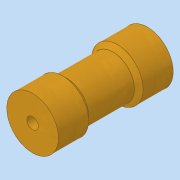
# Autodesk Inventor part: ShaftCoupler
Saved by Autodesk Inventor 2017 (Build 210142000, 142)
## iProperties
Created: 2017-03-06
Part Number: ShaftCoupler
Material: Brass, Soft Yellow, Welded
Document SubType Name: Modeling
Designer: techn
Density: 8.5 g/cm^3
Appearance: Weld - Brass
Author: techn
Autodesk Inventor part; units mm, degrees
ref_plane "YZ Plane" through (0, 0, 0) normal (1, 0, 0) x (0, 1, 0)
ref_plane "XZ Plane" through (0, 0, 0) normal (0, 1, 0) x (-1, 0, 0)
ref_plane "XY Plane" through (0, 0, 0) normal (0, 0, 1) x (1, 0, 0)
sketch "Sketch2" plane through (0, 0, 0) normal (0, 1, 0) x (-1, 0, 0)
  line L0 (0, 0) -> (-4.5, 0)
  line L1 (-4.5, 0) -> (-4.5, -6)
  line L2 (-4.5, -6) -> (0, -6)
  line L3 (0, -6) -> (0, 0)
  line L4 (0, -6) -> (-3.74, -6)
  line L5 (-3.74, -6) -> (-3.74, -14)
  line L6 (-3.74, -14) -> (0, -14)
  line L7 (0, -14) -> (0, -6)
  line L8 (0, -14) -> (-4.5, -14)
  line L9 (-4.5, -14) -> (-4.5, -20)
  line L10 (-4.5, -20) -> (0, -20)
  line L11 (0, -20) -> (0, -14)
  line L12 (0, 0) -> (-1, 0)
  line L13 (-1, 0) -> (-1, -20)
  line L14 (-1, -20) -> (0, -20)
  line L15 (0, -20) -> (0, 0)
  dimension "d0" = 1
  dimension "d1" = 6
  dimension "d2" = 4.5
  dimension "d3" = 20
  dimension "d4" = 6
  dimension "d6" = 4.5
  constraints: 32 end point, 8 parallel, 4 horizontal, 4 perpendicular, 1 point on line
  measures "d0" distance between parallel lines of L3 L13
  measures "d1" distance of L0.end L1.end
  measures "d2" distance between parallel lines of L1 L3
  measures "d3" distance between parallel lines of L0 L10
  measures "d4" distance of L8.end L9.end
  measures "d6" distance between parallel lines of L11 L9
revolve "Revolution1" add sketch "Sketch2" angle 360 about axis through (0, 0, -20) along (0, 0, 1)
revolve "Revolution2" cut sketch "Sketch2" angle 360 about axis through (0, 0, -6) along (0, 0, 1) contours L3 L2 L13 L0 | L7 L6 L13 L2 | L11 L10 L13 L6
chamfer "Chamfer1" distance 0.75 angle 45 2 edges at (-4.5, 0, -14) (-4.5, 0, -6)
equation "\"d4\" = d1"
equation "\"d6\" = d2"
body "Solid1"
